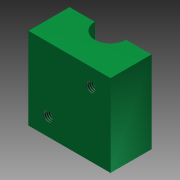
# Autodesk Inventor part: 13_0204_046
Saved by Autodesk Inventor 2012 SP1 (Build 160190100, 190)
## iProperties
Created: 2013-04-08
Part Number: 13_0204_046
Material: Default
Document SubType Name: Modeling
Designer: vogel
Density: 1 g/cm^3
Author: vogel
Autodesk Inventor part; units mm, degrees
ref_plane "YZ Plane" through (0, 0, 0) normal (1, 0, 0) x (0, 1, 0)
ref_plane "XZ Plane" through (0, 0, 0) normal (0, 1, 0) x (-1, 0, 0)
ref_plane "XY Plane" through (0, 0, 0) normal (0, 0, 1) x (1, 0, 0)
sketch "Skizze1" plane through (0, 0, 0) normal (0, 0, 1) x (1, 0, 0)
  line L0 (-10.5, 10.5) -> (10.5, 10.5)
  line L1 (10.5, 10.5) -> (10.5, -10.5)
  line L2 (10.5, -10.5) -> (-10.5, -10.5)
  line L3 (-10.5, -10.5) -> (-10.5, 10.5)
  line L4 (-14.7, 0) -> (14.7, 0) projected
  line L5 (0, -14.7) -> (0, 14.7) projected
  point P0 (0, 0)
  dimension "d0" = 21
  dimension "d1" = 21
  constraints: 8 end point, 2 parallel, 1 horizontal, 1 perpendicular, 2 other
  measures "d0" distance of L2.end L0.start
  measures "d1" distance of L0.start L0.end
extrude "Extrusion1" add sketch "Skizze1" along normal blind 21
sketch "Skizze2" plane through (0, 0, 0) normal (0, 1, 0) x (-1, 0, 0)
  line L0 (14.7, 0) -> (-14.7, 0) projected
  line L1 (0, -4.2) -> (0, 25.2) projected
  line L2 (4, 0) -> (4, 7)
  line L3 (4, 7) -> (9, 7)
  line L4 (9, 7) -> (9, 14)
  line L5 (9, 14) -> (4, 14)
  line L6 (4, 14) -> (4, 21)
  line L7 (-10.5, 21) -> (10.5, 21) projected
  line L8 (10.5, 0) -> (10.5, 21) projected
  line L9 (4, 21) -> (0, 21)
  line L10 (0, 21) -> (0, 0)
  line L11 (4, 0) -> (0, 0)
  dimension "d4" = 8
  dimension "d5" = 18
  dimension "d6" = 7
  dimension "d7" = 7
  constraints: 16 end point, 4 collinear, 3 parallel, 2 point on line, 1 midpoint, 1 perpendicular
  measures "d4" diameter of L2 L1
  measures "d5" diameter of L4 L1
  measures "d6" distance of L2.start L2.end
  measures "d7" distance of L3.end L4.end
revolve "Umdrehung1" cut sketch "Skizze2" angle 360 about axis through (0, 0, -10) along (0, 0, 1) contours L0 L1 L7 L6 L5 L4 L3 L2
sketch "Skizze3" plane through (0, 0, 21) normal (0, 0, 1) x (1, 0, 0)
  line L0 (-10.5, -10.5) -> (-10.5, 10.5) projected
  line L1 (-10.5, 0) -> (10.5, 0)
  line L2 (10.5, 0) -> (10.5, 10.5)
  line L3 (10.5, 10.5) -> (-10.5, 10.5)
  line L4 (-10.5, 10.5) -> (-10.5, 0)
  constraints: 8 end point, 2 parallel, 1 horizontal, 1 midpoint, 1 perpendicular
extrude "Extrusion2" cut sketch "Skizze3" against normal through all
sketch "Skizze4" plane through (0, 0, 0) normal (0, 0, -1) x (-1, 0, 0)
  line L0 (10.5, 0) -> (4, 0) projected
  arc A0 (-4, 0) -> (4, 0) centre (0, 0) ccw projected
  line L1 (-4, 0) -> (-10.5, 0) projected
  arc A1 (-9, 0) -> (9, 0) centre (0, 0) ccw projected
  circle A2 centre (0, 0) radius 9
  constraints: 1 centre point, 1 coincident, 1 concentric
extrude "Extrusion3" cut sketch "Skizze4" against normal up to surface (7 mm away) contours A1 L1 A0 L0
sketch "Skizze5" plane through (-10.5, -10.5, 0) normal (0, -1, 0) x (1, 0, 0)
  point P0 (5, 4.5)
hole "Bohrung1" at (-5.5, -10.5, 4.5) direction (0, 1, 0) diameter 2.459 depth 7.5 tip angle 120 thread size "M3x0.5" class "6H" standard "ISO Metric profile"
sketch "Skizze6" plane through (-10.5, -10.5, 0) normal (0, -1, 0) x (1, 0, 0)
  point P0 (16, 16.5)
hole "Bohrung3" at (5.5, -10.5, 16.5) direction (0, 1, 0) diameter 2.459 depth 7.5 tip angle 120 thread size "M3x0.5" class "6H" standard "ISO Metric profile"
